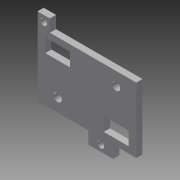
# Autodesk Inventor part: hook mount plate 2
Saved by Autodesk Inventor 2013 (Build 170138000, 138)
## iProperties
Created: 2013-01-27
Part Number: hook mount plate 2
Material: Steel
Document SubType Name: Sheet Metal
Designer: Arpan
Density: 7.85 g/cm^3
Sheet Metal Rule: Default
Mass: 318.43 g
Surface Area: 168.381 cm^2
Volume: 40.5643 cm^3
Author: Arpan
Autodesk Inventor part; units mm, degrees
ref_plane "YZ Plane" through (0, 0, 0) normal (1, 0, 0) x (0, 1, 0)
ref_plane "XZ Plane" through (0, 0, 0) normal (0, 1, 0) x (-1, 0, 0)
ref_plane "XY Plane" through (0, 0, 0) normal (0, 0, 1) x (1, 0, 0)
sketch "Sketch1" plane through (0, 0, 0) normal (0, 0, 1) x (1, 0, 0)
  line L0 (80.7, -46.515) -> (80.7, -60.485)
  line L1 (80.7, -60.485) -> (55.3, -60.485)
  line L2 (55.3, -60.485) -> (55.3, -46.515)
  line L3 (55.3, -46.515) -> (80.7, -46.515)
  line L4 (-4.699, -6.5024) -> (20.701, -6.5024)
  line L5 (20.701, -6.5024) -> (20.701, -20.4724)
  line L6 (20.701, -20.4724) -> (-4.699, -20.4724)
  line L7 (-4.699, -20.4724) -> (-4.699, -6.5024)
  circle A0 centre (8, -53.5) radius 4.15
  circle A1 centre (68, -13.5) radius 4.15
  line L8 (25.3, 0) -> (-12.7, 0)
  line L9 (-12.7, 0) -> (-12.7, -67)
  line L10 (-12.7, -67) -> (41.175, -67)
  line L11 (66.575, -67) -> (88.7, -67)
  line L12 (88.7, -67) -> (88.7, 0)
  line L13 (88.7, 0) -> (50.7, 0)
  line L14 (66.575, -67) -> (41.175, -67)
  line L15 (25.3, 0) -> (50.7, 0)
  line L16 (38, -67) -> (52.2875, -67)
  line L17 (52.2875, -79.7) -> (39.5875, -79.7)
  line L18 (39.5875, -79.7) -> (39.5875, -67)
  line L19 (52.2875, -79.7) -> (64.9875, -79.7)
  line L20 (64.9875, -79.7) -> (64.9875, -67)
  circle A2 centre (52.2875, -73.35) radius 3.3782
  line L21 (88.7, 0) -> (76, 0)
  line L22 (-12.7, 0) -> (-12.7, 12.7)
  line L23 (-12.7, 12.7) -> (0, 12.7)
  line L24 (0, 12.7) -> (0, 0)
  line L25 (-6.35, 0) -> (-6.35, 6.35)
  circle A3 centre (-6.35, 6.35) radius 3.3782
  point P0 (82.35, 0)
  dimension "d0" = 14.2875
  dimension "d3" = 12.7
  dimension "d5" = 6.7564
  dimension "d6" = 12.7
  dimension "d11" = 12.7
  dimension "d12" = 12.7
  dimension "d13" = 6.7564
  measures "d0" distance of L16.start L16.end
  measures "d3" distance of L17.start L17.end
  measures "d5" diameter of A2
  measures "d6" distance of L12.end L21.end
  measures "d11" distance of L8.end L22.end
  measures "d12" distance of L22.end L23.end
  measures "d13" diameter of A3
extrude "Plate2" add sketch "Sketch1" along normal blind 6.35
equation "\"BendRadius\" = Thickness"
equation "\"BendReliefWidth\" = Thickness"
equation "\"BendReliefDepth\" = 0.5 * Thickness"
equation "\"CornerReliefSize\" = 4 * Thickness"
equation "\"MinimumRemnant\" = 2 * Thickness"
equation "\"TransitionRadius\" = BendRadius"
equation "\"JacobiRadiusSize\" = BendRadius"
equation "\"GapSize\" = Thickness"
equation "\"d9\" = BendRadius"
equation "\"d10\" = BendRadius"
equation "\"Thickness\" = 6.35"
body "Solid2"
